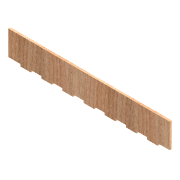
# Autodesk Inventor part: achterzijde elektrobox v2
Saved by Autodesk Inventor 2020.3 (Build 243373000, 373)
## iProperties
Created: 2020-11-26
Part Number: achterzijde elektrobox v2
Material: Wood (Birch)
Document SubType Name: Sheet Metal
Designer: Svend
Density: 0.55 g/cm^3
Sheet Metal Rule: Default_mm
Appearance: Birch - Natural Polished
Author: Svend
Autodesk Inventor part; units mm, degrees
ref_plane "YZ Plane" through (0, 0, 0) normal (1, 0, 0) x (0, 1, 0)
ref_plane "XZ Plane" through (0, 0, 0) normal (0, 1, 0) x (-1, 0, 0)
ref_plane "XY Plane" through (0, 0, 0) normal (0, 0, 1) x (1, 0, 0)
ref_plane "Work Plane1" through (0, 0, 0) normal (0, 0, 1) x (1, 0, 0)
sketch "Sketch1" plane through (0, 0, 0) normal (0, 0, 1) x (1, 0, 0)
  line L0 (-34, 6) -> (-34, 0)
  line L1 (-34, 0) -> (0, 0)
  line L2 (0, 0) -> (0, 6)
  line L3 (0, 6) -> (-34, 6)
  line L4 (0, 6) -> (30, 6)
  line L5 (0, 0) -> (0, 6)
  line L6 (30, 0) -> (0, 0)
  line L7 (30, 0) -> (30, 6)
  line L8 (30, 6) -> (30, 0)
  line L9 (30, 0) -> (60, 0)
  line L10 (60, 0) -> (60, 6)
  line L11 (60, 6) -> (30, 6)
  line L12 (60, 6) -> (90, 6)
  line L13 (60, 0) -> (60, 6)
  line L14 (90, 0) -> (60, 0)
  line L15 (90, 0) -> (90, 6)
  line L16 (90, 6) -> (90, 0)
  line L17 (90, 0) -> (120, 0)
  line L18 (120, 0) -> (120, 6)
  line L19 (120, 6) -> (90, 6)
  line L20 (120, 6) -> (150, 6)
  line L21 (120, 0) -> (120, 6)
  line L22 (150, 0) -> (120, 0)
  line L23 (150, 0) -> (150, 6)
  line L24 (150, 6) -> (150, 0)
  line L25 (150, 0) -> (180, 0)
  line L26 (180, 0) -> (180, 6)
  line L27 (180, 6) -> (150, 6)
  line L28 (180, 6) -> (210, 6)
  line L29 (180, 6) -> (210, 6)
  line L30 (180, 0) -> (180, 6)
  line L31 (210, 0) -> (180, 0)
  line L32 (210, 0) -> (210, 6)
  line L33 (240, 0) -> (240, 6)
  line L34 (240, 6) -> (210, 6)
  line L35 (210, 6) -> (210, 0)
  line L36 (210, 0) -> (240, 0)
  line L37 (240, 6) -> (270, 6)
  line L38 (240, 0) -> (240, 6)
  line L39 (270, 0) -> (240, 0)
  line L40 (270, 0) -> (270, 6)
  line L41 (300, 0) -> (300, 6)
  line L42 (300, 6) -> (270, 6)
  line L43 (270, 6) -> (270, 0)
  line L44 (270, 0) -> (300, 0)
  line L45 (300, 6) -> (330, 6)
  line L46 (300, 0) -> (300, 6)
  line L47 (330, 0) -> (300, 0)
  line L48 (330, 0) -> (330, 6)
  line L49 (360, 0) -> (360, 6)
  line L50 (360, 6) -> (330, 6)
  line L51 (330, 6) -> (330, 0)
  line L52 (330, 0) -> (360, 0)
  line L53 (360, 6) -> (390, 6)
  line L54 (360, 0) -> (360, 6)
  line L55 (390, 0) -> (360, 0)
  line L56 (390, 0) -> (390, 6)
  line L57 (424, 0) -> (424, 6)
  line L58 (424, 6) -> (390, 6)
  line L59 (390, 6) -> (390, 0)
  line L60 (390, 0) -> (424, 0)
  line L61 (-34, 6) -> (424, 6)
  line L62 (424, 6) -> (424, 76)
  line L63 (424, 76) -> (-34, 76)
  line L64 (-34, 76) -> (-34, 6)
  line L65 (401, 57.7) -> (300, 57.7)
  dimension "d0" = 70
  measures "d0" distance of L61.end L62.end
extrude "Plate1" add sketch "Sketch1" along normal blind 6 contours L64 L63 L62 L58 L53 L50 L45 L42 L37 L34 L28 L27 L20 L19 L12 L11 L4 L3 | L4 L7 L6 L2 | L12 L15 L14 L10 | L56 L55 L49 L53 | L20 L23 L22 L18 | L48 L47 L41 L45 | L28 L32 L31 L26 | L40 L39 L33 L37
equation "\"d1\" = Thickness"
equation "\"BendRadius\" = Thickness"
equation "\"BendReliefWidth\" = Thickness"
equation "\"BendReliefDepth\" = 0.5 * Thickness"
equation "\"CornerReliefSize\" = 4 * Thickness"
equation "\"MinimumRemnant\" = 2 * Thickness"
equation "\"TransitionRadius\" = BendRadius"
equation "\"JacobiRadiusSize\" = BendRadius"
equation "\"GapSize\" = Thickness"
equation "\"Thickness\" = 6"
body "Solid1"
